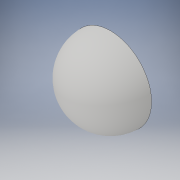
# Autodesk Inventor part: gabung sama tutup lampu
Saved by Autodesk Inventor 2019.5 (Build 235369000, 369)
## iProperties
Created: 2022-10-11
Part Number: gabung sama tutup lampu
Material: Generic
Document SubType Name: Modeling
Designer: ASUS
Density: 1 g/cm^3
Appearance: Default
Author: ASUS
Autodesk Inventor part; units mm, degrees
ref_plane "YZ Plane" through (0, 0, 0) normal (1, 0, 0) x (0, 1, 0)
ref_plane "XZ Plane" through (0, 0, 0) normal (0, 1, 0) x (-1, 0, 0)
ref_plane "XY Plane" through (0, 0, 0) normal (0, 0, 1) x (1, 0, 0)
sketch "Sketch1" plane through (0, 0, 0) normal (0, 0, 1) x (1, 0, 0)
  circle A0 centre (17.2364, 8.0687) radius 15
  line L0 (17.2364, 23.0687) -> (17.2364, -6.9313)
  point P0 (0, 0)
  dimension "d0" = 30
  constraints: 2 end point, 2 point on circle, 1 centre point
  measures "d0" diameter of A0
revolve "Revolution1" add sketch "Sketch1" angle 180 about axis through (17.2364, 23.0687, 0) along (0, 1, 0) picked at (12.2729, 8.6714) contours L0 A0
shell "Shell1" thickness 1 removed faces 2 at (8.7527, 8.2439, 0) at (25.7202, 8.2439, 0)
body "Solid1"
